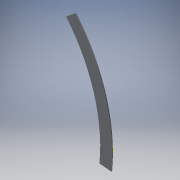
# Autodesk Inventor part: externalSupportRear1
Saved by Autodesk Inventor 2019 (Build 230136000, 136)
## iProperties
Created: 2019-01-12
Part Number: externalSupportRear1
Material: Wood (Cherry)
Document SubType Name: Modeling
Designer: gaincarlo
Density: 0.63 g/cm^3
Appearance: Cherry - Natural Low Gloss
Author: gaincarlo
Autodesk Inventor part; units mm, degrees
ref_plane "YZ Plane" through (0, 0, 0) normal (1, 0, 0) x (0, 1, 0)
ref_plane "XZ Plane" through (0, 0, 0) normal (0, 1, 0) x (-1, 0, 0)
ref_plane "Work Plane1" through (0, 0, 0) normal (0, 0, 1) x (1, 0, 0)
sketch "Sketch1" plane through (0, 0, 0) normal (0, 0, 1) x (1, 0, 0)
  line L0 (-507.2437, -32.9396) -> (89.7639, -92.7893) construction
  arc A0 (22.3112, -84.0063) -> (-126.1247, 408.4057) centre (-651.3316, -18.4949) ccw construction
  line L1 (-74.7461, 453.0192) -> (-539.2143, 73.1912) construction
  line L2 (46.1596, 196.9837) -> (49.0458, 187.4093) construction
  arc A1 (75.0276, -91.312) -> (47.6027, 192.1965) centre (-651.3316, -18.4949) ccw
  arc A2 (47.6027, 192.1965) -> (-86.2286, 443.6292) centre (-651.3316, -18.4949) ccw
  arc A3 (22.1136, -86.0074) -> (-127.3954, 409.9642) centre (-651.3316, -18.4949) ccw
  line L3 (75.0276, -91.312) -> (22.1136, -86.0074)
  line L4 (-86.2286, 443.6292) -> (-127.3954, 409.9642)
  point P0 (0, 0)
  constraints: 7 point on circle, 4 end point, 3 centre point, 3 coincident, 3 point on line, 1 collinear, 1 midpoint
extrude "Extrusion1" add sketch "Sketch1" along normal blind 4
body "Solid1"
